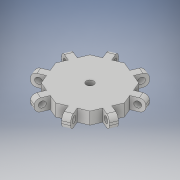
# Autodesk Inventor part: Hex_Center
Saved by Autodesk Inventor 2019 (Build 230136000, 136)
## iProperties
Created: 2019-11-16
Part Number: Hex_Center
Material: Generic
Document SubType Name: Modeling
Designer: Jorian Brusind
Density: 1 g/cm^3
Appearance: Default
Author: Jorian Brusind
Autodesk Inventor part; units mm, degrees
ref_plane "YZ Plane" through (0, 0, 0) normal (1, 0, 0) x (0, 1, 0)
ref_plane "XZ Plane" through (0, 0, 0) normal (0, 1, 0) x (-1, 0, 0)
ref_plane "XY Plane" through (0, 0, 0) normal (0, 0, 1) x (1, 0, 0)
sketch "Sketch1" plane through (0, 0, 0) normal (0, 1, 0) x (-1, 0, 0)
  line L0 (14.1421, 0) -> (10, -10)
  line L1 (10, -10) -> (0, -14.1421)
  line L2 (0, -14.1421) -> (-10, -10)
  line L3 (-10, -10) -> (-14.1421, 0)
  line L4 (-14.1421, 0) -> (-10, 10)
  line L5 (-10, 10) -> (0, 14.1421)
  line L6 (0, 14.1421) -> (10, 10)
  line L7 (10, 10) -> (14.1421, 0)
  point P0 (0, 0)
  point P1 (0, 0)
  dimension "d36" = 10
  dimension "d37" = 10
  constraints: 16 end point, 1 coincident, 17 other
  measures "d36" vertical distance of L0.start L0.end
  measures "d37" vertical distance of L6.end L0.start
extrude "Extrusion1" add sketch "Sketch1" along normal blind 5
sketch "Sketch2" plane through (0, 5, 0) normal (0, 1, 0) x (1, 0, 0)
  circle A0 centre (0, 0) radius 1.5
  dimension "d4" = 3
  constraints: 1 centre point, 1 coincident
  measures "d4" diameter of A0
extrude "Extrusion2" cut sketch "Sketch2" against normal blind 5
sketch "Sketch3" plane through (10, 0, 10) normal (0.3826834, 0, 0.9238795) x (0.9238795, 0, -0.3826834)
  line L0 (-10.8239, 5) -> (-6.8239, 5)
  line L1 (0, 5) -> (-10.8239, 5) projected
  line L2 (0, 5) -> (-4, 5)
  line L3 (-6.8239, 5) -> (-5.3239, 5)
  line L4 (-5.3239, 5) -> (-5.3239, 0)
  line L5 (-5.3239, 0) -> (-6.8239, 0)
  line L6 (-6.8239, 0) -> (-6.8239, 5)
  line L7 (-10.8239, 0) -> (0, 0) projected
  line L8 (-4, 5) -> (-5.5, 5)
  line L9 (-5.5, 5) -> (-5.5, 0)
  line L10 (-5.5, 0) -> (-4, 0)
  line L11 (-4, 0) -> (-4, 5)
  dimension "d21" = 4
  dimension "d22" = 4
  dimension "d23" = 1.5
  dimension "d24" = 5
  dimension "d25" = 1.5
  constraints: 20 end point, 4 parallel, 3 point on line, 2 horizontal, 2 perpendicular
  measures "d21" distance of L0.start L0.end
  measures "d22" distance of L1.start L2.end
  measures "d23" distance of L4.end L5.end
  measures "d24" distance of L3.end L4.end
  measures "d25" distance of L10.end L9.end
extrude "Extrusion5" add sketch "Sketch3" along normal blind 5
sketch "Sketch5" plane through (6.3045, 0, 11.5307) normal (0.9238795, 0, -0.3826834) x (-0.3826834, 0, -0.9238795)
  line L0 (0, 0) -> (-5, 0) projected
  line L1 (-5, 0) -> (-2.5, 0)
  line L2 (-2.5, 0) -> (-2.5, 2.5)
  circle A0 centre (-2.5, 2.5) radius 1.25
  point P0 (13.0656, 0)
  dimension "d28" = 2.5
  dimension "d29" = 2.5
  constraints: 4 end point, 1 centre point, 1 coincident, 1 midpoint, 1 vertical
  measures "d28" distance of L1.end L2.end
  measures "d29" diameter of A0
extrude "Extrusion6" cut sketch "Sketch5" against normal blind 8
fillet "Fillet1" radius 2 2 edges at (6.9134, 0, 16.6905) (6.9134, 5, 16.6905)
pattern_circular "Circular Pattern2" count 8 over 360 about axis through (0, 5, 0) along (0, -1, 0) of "Extrusion6", "Extrusion5", "Fillet1"
body "Solid1"
